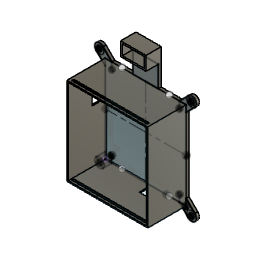
PCBCase (Autodesk Fusion 360 design; units mm, degrees)
Autodesk Fusion 360 part; units mm, degrees
sketch "Sketch1" plane through (0, 0, 0) normal (0, 1, 0) x (1, 0, 0)
  line L0 (0, 0) -> (95, 0)
  line L1 (95, 0) -> (95, -103)
  line L2 (95, -103) -> (7.75, -103)
  line L3 (0, -95.25) -> (0, 0)
  line L4 (0, -103) -> (7.75, -103)
  line L5 (7.75, -103) -> (7.75, -95.25)
  circle A0 centre (7.75, -95.25) radius 2
  line L6 (0, -103) -> (7.75, -103)
  line L7 (0, -103) -> (0, -95.25)
  line L8 (0, -95.25) -> (-10.6066, -105.8566)
  line L9 (7.75, -103) -> (-2.8566, -113.6066)
  line L10 (7.75, -103) -> (19.75, -103) construction
  line L11 (-10.6066, -105.8566) -> (-2.8566, -113.6066)
  circle A1 centre (-6.7316, -109.7316) radius 5.5
  line L12 (95, -51.5) -> (0, -51.5)
  line L13 (47.5, 0) -> (47.5, -103)
  circle A2 centre (-6.7316, -109.7316) radius 2.5
  circle A3 centre (-6.7316, 6.7316) radius 5.5
  circle A4 centre (7.75, -7.75) radius 2
  line L14 (7.75, 0) -> (19.75, 0) construction
  line L15 (0, -7.75) -> (-10.6066, 2.8566)
  line L16 (7.75, 0) -> (-2.8566, 10.6066)
  line L17 (0, 0) -> (0, -7.75)
  line L18 (7.75, 0) -> (7.75, -7.75)
  line L19 (0, 0) -> (7.75, 0)
  circle A5 centre (-6.7316, 6.7316) radius 2.5
  line L20 (0, 0) -> (7.75, 0)
  line L21 (-10.6066, 2.8566) -> (-2.8566, 10.6066)
  line L22 (87.25, -103) -> (75.25, -103) construction
  circle A6 centre (87.25, -95.25) radius 2
  line L23 (87.25, -103) -> (87.25, -95.25)
  line L24 (95, -95.25) -> (105.6066, -105.8566)
  line L25 (105.6066, -105.8566) -> (97.8566, -113.6066)
  circle A7 centre (101.7316, -109.7316) radius 5.5
  line L26 (95, -103) -> (87.25, -103)
  circle A8 centre (101.7316, -109.7316) radius 2.5
  line L27 (95, -103) -> (87.25, -103)
  line L28 (105.6066, 2.8566) -> (97.8566, 10.6066)
  line L29 (87.25, 0) -> (87.25, -7.75)
  line L30 (87.25, 0) -> (75.25, 0) construction
  line L31 (95, 0) -> (87.25, 0)
  line L32 (95, -103) -> (95, -95.25)
  line L33 (95, -7.75) -> (105.6066, 2.8566)
  line L34 (95, 0) -> (95, -7.75)
  line L35 (95, 0) -> (87.25, 0)
  line L36 (87.25, -103) -> (97.8566, -113.6066)
  circle A9 centre (101.7316, 6.7316) radius 2.5
  circle A10 centre (87.25, -7.75) radius 2
  line L37 (87.25, 0) -> (97.8566, 10.6066)
  circle A11 centre (101.7316, 6.7316) radius 5.5
  line L38 (47.5, -103) -> (62.4, -103)
  line L39 (62.4, -103) -> (32.6, -103)
  line L40 (32.6, -103) -> (32.6, -128)
  line L41 (32.6, -128) -> (62.4, -128)
  line L42 (62.4, -128) -> (62.4, -103)
  point P0 (95, 0)
  point P1 (95, -51.5)
  point P2 (95, 0)
  dimension "d1" = 95
  dimension "d2" = 103
  dimension "d3" = 7.75
  dimension "d4" = 7.75
  dimension "d5" = 4
  dimension "d6" = 7.75
  dimension "d7" = 7.75
  dimension "d8" = 15
  dimension "d9" = 135
  dimension "d10" = 135
  dimension "d11" = 15
  dimension "d12" = 11
  dimension "d17" = 5
  dimension "d58" = 14.9
  dimension "d59" = 29.8
  dimension "d60" = 25
  constraint horizontal L0
  constraint vertical L1
  constraint horizontal L2
  constraint vertical L3
  constraint coincident L0.start L3.end
  constraint perpendicular L3 L4
  constraint perpendicular L2 L5
  constraint coincident L5.end A0.centre
  constraint perpendicular L3 L6
  constraint perpendicular L4 L7
  constraint horizontal L10
  constraint midpoint L11 A1.centre
  constraint midpoint L1 P1
  constraint coincident L3 L12.end
  constraint perpendicular L3 L12
  constraint midpoint L0 L13.start
  constraint coincident L2 L13.end
  constraint perpendicular L2 L13
  constraint concentric A1 A2
  constraint symmetric L4.start L12 L0.start
  constraint symmetric L2.end L12 L14.start
  constraint symmetric L5.end L12 A4.centre
  constraint symmetric A0 L12 A4
  constraint symmetric L3.start L12 L15.start
  constraint symmetric L8.end L12 L15.end
  constraint symmetric L9.end L12 L16.end
  constraint symmetric L10.end L12 L14.end
  constraint symmetric A1 L12 A3
  constraint symmetric L12 A2 A5
  constraint symmetric L0.start L13 P2
  constraint symmetric L4.start L13 L1.end
  constraint symmetric L2.end L13 L22.start
  constraint symmetric L5.end L13 A6.centre
  constraint symmetric A0 L13 A6
  constraint symmetric L3.start L13 L24.start
  constraint symmetric L8.end L13 L24.end
  constraint symmetric L9.end L13 L25.end
  constraint symmetric L10.end L13 L22.end
  constraint symmetric A1 L13 A7
  constraint symmetric L12.end L13 P1
  constraint symmetric L13 A2 A8
  constraint symmetric L13 L15.start L33.start
  constraint symmetric L13 L16.end L28.end
  constraint symmetric L13 L15.end L28.start
  constraint symmetric L13 L14.start L29.start
  constraint symmetric L13 A4.centre L29.end
  constraint symmetric L13 L14.end L30.end
  constraint symmetric L13 L0.start P2
  constraint symmetric L13 A3 A11
  constraint symmetric L13 A4 A10
  constraint symmetric L13 A5 A9
  constraint perpendicular L13 L38
  constraint horizontal L39
  constraint vertical L40
  constraint horizontal L41
  constraint vertical L42
  measures "d1" distance of L0.start P0
  measures "d2" distance of L0.start L4.start
  measures "d3" distance of L4.start L2.end
  measures "d4" distance of L2.end L5.end
  measures "d5" diameter of A0
  measures "d6" distance of L4.start L2.end
  measures "d7" distance of L4.start L3.start
  measures "d8" distance of L3.start L8.end
  measures "d9" angle of L3 L8
  measures "d10" angle of L9 L10
  measures "d11" distance of L2.end L9.end
  measures "d12" diameter of A1
  measures "d17" diameter of A2
  measures "d58" distance of L13.end L38.end
  measures "d59" distance of L38.end L39.end
  measures "d60" distance of L38.end L41.end
extrude "Extrude1" add sketch "Sketch1" along normal blind 3.5 contours L0 L3 A3 L15 L16 L17 L19 L20 | L0 L3 L12 L13 L17 L19 L20 | L0 L1 L12 L13 L31 L34 L35 | A3 L15 L16 A5 L21 | A3 L15 L16 A5 L21 | L2 L3 L4 L6 L7 L12 L13 L39 | L0 L1 L31 L33 L34 L35 L37 A11 | L1 L2 L12 L13 L26 L27 L32 L38 L39 | L4 L6 L7 L8 L9 A1 | L28 L33 A9 L37 A11 | L28 L33 A9 L37 A11 | L8 L9 L11 A1 A2 | L8 L9 L11 A1 A2 | L1 L2 L24 A7 L26 L27 L32 L36 | L24 L25 A7 A8 L36 | L24 L25 A7 A8 L36
sketch "Sketch2" plane through (0, 0, 0) normal (0, -1, 0) x (1, 0, 0)
  circle A0 centre (7.75, 7.75) radius 2
  circle A1 centre (87.25, 7.75) radius 2
  circle A2 centre (-6.7316, -6.7316) radius 2.5
  circle A3 centre (101.7316, -6.7316) radius 2.5
  circle A4 centre (87.25, 95.25) radius 2
  circle A5 centre (101.7316, 109.7316) radius 2.5
  circle A6 centre (7.75, 95.25) radius 2
  circle A7 centre (-6.7316, 109.7316) radius 2.5
  line L0 (105.2759, -2.5259) -> (95, 7.75)
  line L1 (95, 7.75) -> (95, 95.25)
  line L2 (95, 95.25) -> (105.2759, 105.5259)
  arc A8 (105.2759, 105.5259) -> (97.5259, 113.2759) centre (101.7316, 109.7316) ccw
  line L3 (97.5259, 113.2759) -> (87.25, 103)
  line L4 (87.25, 103) -> (7.75, 103)
  line L5 (7.75, 103) -> (-2.5259, 113.2759)
  arc A9 (-2.5259, 113.2759) -> (-10.2759, 105.5259) centre (-6.7316, 109.7316) ccw
  line L6 (-10.2759, 105.5259) -> (0, 95.25)
  line L7 (0, 95.25) -> (0, 7.75)
  line L8 (0, 7.75) -> (-10.2759, -2.5259)
  arc A10 (-10.2759, -2.5259) -> (-2.5259, -10.2759) centre (-6.7316, -6.7316) ccw
  line L9 (-2.5259, -10.2759) -> (7.75, 0)
  line L10 (7.75, 0) -> (87.25, 0)
  line L11 (87.25, 0) -> (97.5259, -10.2759)
  arc A11 (97.5259, -10.2759) -> (105.2759, -2.5259) centre (101.7316, -6.7316) ccw
  line L12 (47.5, 103) -> (47.5, 0) construction
  line L13 (0, 51.5) -> (95, 51.5) construction
  line L14 (0, 0) -> (1.5, 0)
  line L15 (1.5, 0) -> (1.5, 103)
  line L16 (1.5, 103) -> (0, 103)
  line L17 (0, 103) -> (0, 0)
  line L18 (95, 103) -> (95, 0)
  line L19 (93.5, 0) -> (93.5, 103)
  line L20 (93.5, 103) -> (95, 103)
  line L21 (95, 0) -> (93.5, 0)
  line L22 (0, 103) -> (95, 103)
  line L23 (95, 103) -> (95, 101.5)
  line L24 (95, 101.5) -> (0, 101.5)
  line L25 (0, 101.5) -> (0, 103)
  line L26 (95, 1.5) -> (0, 1.5)
  line L27 (0, 0) -> (95, 0)
  line L28 (95, 0) -> (95, 1.5)
  line L29 (0, 1.5) -> (0, 0)
  dimension "d22" = 1.5
  dimension "d23" = 103
  dimension "d24" = 95
  dimension "d25" = 1.5
  constraint midpoint L4 L12.start
  constraint midpoint L10 L12.end
  constraint midpoint L7 L13.start
  constraint midpoint L1 L13.end
  constraint horizontal L14
  constraint vertical L15
  constraint horizontal L16
  constraint vertical L17
  constraint coincident L14.start L17.end
  constraint symmetric L12 L14.start L18.end
  constraint symmetric L12 L14.end L19.start
  constraint symmetric L12 L15.end L19.end
  constraint symmetric L12 L16.end L18.start
  constraint horizontal L22
  constraint vertical L23
  constraint horizontal L24
  constraint vertical L25
  constraint symmetric L13 L16.end L14.start
  constraint symmetric L13 L18.start L18.end
  constraint symmetric L13 L23.end L26.start
  constraint symmetric L13 L24.end L26.end
  measures "d22" distance of L14.start L14.end
  measures "d23" distance of L14.start L16.end
  measures "d24" distance of L16.end L18.start
  measures "d25" distance of L16.end L24.end
extrude "Extrude2" add sketch "Sketch2" along normal blind 45 contours L1 L18 L19 L24 L26 | L18 L19 L21 L26 L27 L28 | L10 L15 L19 L26 L27 | L18 L19 L20 L22 L23 L24 | L4 L15 L19 L22 L24 | L7 L15 L17 L24 L26 | L14 L15 L17 L26 L27 L29 | L15 L16 L17 L22 L24 L25
sketch "Sketch3" plane through (0, 0, 0) normal (0, 0, -1) x (1, 0, 0)
  line L0 (7.75, 0) -> (7.75, -3.5)
  line L1 (7.75, -3.5) -> (87.25, -3.5)
  line L2 (87.25, -3.5) -> (87.25, 0)
  line L3 (87.25, 0) -> (95, 0)
  line L4 (95, 0) -> (95, 45)
  line L5 (95, 45) -> (0, 45)
  line L6 (0, 45) -> (0, 0)
  line L7 (0, 0) -> (7.75, 0)
  line L8 (0, 45) -> (0, 42.5)
  line L9 (0, 42.5) -> (3, 42.5)
  line L10 (3, 42.5) -> (92, 42.5)
  line L11 (92, 42.5) -> (92, 40)
  line L12 (92, 40) -> (3, 40)
  line L13 (3, 40) -> (3, 42.5)
  dimension "d28" = 2.5
  dimension "d29" = 3
  dimension "d30" = 89
  dimension "d31" = 2.5
  constraint coincident L5.end L6.start
  constraint perpendicular L5 L8
  constraint perpendicular L8 L9
  constraint horizontal L10
  constraint vertical L11
  constraint horizontal L12
  constraint vertical L13
  measures "d28" distance of L5.end L8.end
  measures "d29" distance of L8.end L9.end
  measures "d30" distance of L9.end L10.end
  measures "d31" distance of L9.end L12.end
extrude "Extrude3" cut sketch "Sketch3" against normal blind 156 contours L10 L11 L12 L13
sketch "Sketch4" plane through (0, 0, 0) normal (0, -1, 0) x (1, 0, 0)
  circle A0 centre (7.75, 95.25) radius 2
  circle A1 centre (87.25, 95.25) radius 2
  circle A2 centre (87.25, 7.75) radius 2
  circle A3 centre (7.75, 7.75) radius 2
  line L0 (93.5, 1.5) -> (93.5, 101.5)
  line L1 (93.5, 101.5) -> (1.5, 101.5)
  line L2 (1.5, 101.5) -> (1.5, 1.5)
  line L3 (1.5, 1.5) -> (93.5, 1.5)
extrude "Extrude5" add sketch "Sketch1" along normal blind 3.5 contours L0 L3 L12 L13 L17 L19 L20
sketch "Sketch5" plane through (0, 3.5, 0) normal (0, 1, 0) x (-1, 0, 0)
  circle A0 centre (-7.75, 95.25) radius 2
  circle A1 centre (6.7316, 109.7316) radius 2.5
  circle A2 centre (-101.7316, -6.7316) radius 2.5
  circle A3 centre (-101.7316, 109.7316) radius 2.5
  circle A4 centre (-87.25, 95.25) radius 2
  circle A5 centre (-7.75, 7.75) radius 2
  circle A6 centre (6.7316, -6.7316) radius 2.5
  circle A7 centre (-87.25, 7.75) radius 2
  line L0 (-95, 7.75) -> (-105.2759, -2.5259)
  arc A8 (-105.2759, -2.5259) -> (-97.5259, -10.2759) centre (-101.7316, -6.7316) ccw
  line L1 (-97.5259, -10.2759) -> (-87.25, 0)
  line L2 (-87.25, 0) -> (-7.75, 0)
  line L3 (-7.75, 0) -> (2.5259, -10.2759)
  arc A9 (2.5259, -10.2759) -> (10.2759, -2.5259) centre (6.7316, -6.7316) ccw
  line L4 (10.2759, -2.5259) -> (0, 7.75)
  line L5 (0, 7.75) -> (0, 95.25)
  line L6 (0, 95.25) -> (10.2759, 105.5259)
  arc A10 (10.2759, 105.5259) -> (2.5259, 113.2759) centre (6.7316, 109.7316) ccw
  line L7 (2.5259, 113.2759) -> (-7.75, 103)
  line L8 (-7.75, 103) -> (-87.25, 103)
  line L9 (-87.25, 103) -> (-97.5259, 113.2759)
  arc A11 (-97.5259, 113.2759) -> (-105.2759, 105.5259) centre (-101.7316, 109.7316) ccw
  line L10 (-105.2759, 105.5259) -> (-95, 95.25)
  line L11 (-95, 95.25) -> (-95, 7.75)
  line L12 (25, 66.4) -> (41.2, 66.4)
  line L13 (41.2, 66.4) -> (41.2, 36.6)
  line L14 (41.2, 36.6) -> (25, 36.6)
  line L15 (25, 36.6) -> (25, 66.4)
  dimension "d48" = 16.2
  dimension "d49" = 29.8
  constraint horizontal L12
  constraint vertical L13
  constraint horizontal L14
  constraint vertical L15
  measures "d48" distance of L12.start L12.end
  measures "d49" distance of L12.start L14.end
extrude "Extrude8" add sketch "Sketch1" along normal blind 3.5 contours L2 L38 L39 L40 L41 L42
sketch "Sketch7" plane through (0, 3.5, 0) normal (0, 1, 0) x (-1, 0, 0)
  line L0 (-62.4, 128) -> (-62.4, 103)
  line L1 (-7.75, 103) -> (-32.6, 103)
  line L2 (-32.6, 103) -> (-32.6, 128)
  line L3 (-32.6, 128) -> (-62.4, 128)
  line L4 (-62.4, 128) -> (-32.6, 128)
  line L5 (-32.6, 128) -> (-32.6, 144.2)
  line L6 (-32.6, 144.2) -> (-62.4, 144.2)
  line L7 (-62.4, 144.2) -> (-62.4, 128)
  circle A0 centre (6.7316, -6.7316) radius 2.5
  circle A1 centre (-7.75, 7.75) radius 2
  line L8 (-87.25, 0) -> (-7.75, 0)
  line L9 (-7.75, 0) -> (2.5259, -10.2759)
  arc A2 (2.5259, -10.2759) -> (10.2759, -2.5259) centre (6.7316, -6.7316) ccw
  line L10 (10.2759, -2.5259) -> (0, 7.75)
  line L11 (0, 7.75) -> (0, 95.25)
  line L12 (0, 95.25) -> (10.2759, 105.5259)
  arc A3 (10.2759, 105.5259) -> (2.5259, 113.2759) centre (6.7316, 109.7316) ccw
  line L13 (2.5259, 113.2759) -> (-7.75, 103)
  line L14 (-62.4, 103) -> (-87.25, 103)
  line L15 (-87.25, 103) -> (-97.5259, 113.2759)
  arc A4 (-97.5259, 113.2759) -> (-105.2759, 105.5259) centre (-101.7316, 109.7316) ccw
  line L16 (-105.2759, 105.5259) -> (-95, 95.25)
  line L17 (-95, 95.25) -> (-95, 7.75)
  line L18 (-95, 7.75) -> (-105.2759, -2.5259)
  arc A5 (-105.2759, -2.5259) -> (-97.5259, -10.2759) centre (-101.7316, -6.7316) ccw
  line L19 (-97.5259, -10.2759) -> (-87.25, 0)
  circle A6 centre (-7.75, 95.25) radius 2
  circle A7 centre (-87.25, 7.75) radius 2
  circle A8 centre (-87.25, 95.25) radius 2
  circle A9 centre (6.7316, 109.7316) radius 2.5
  circle A10 centre (-101.7316, 109.7316) radius 2.5
  circle A11 centre (-101.7316, -6.7316) radius 2.5
  dimension "d63" = 29.8
  dimension "d64" = 16.2
  constraint horizontal L4
  constraint vertical L5
  constraint horizontal L6
  constraint vertical L7
  constraint coincident L0.start L3.end
  measures "d63" distance of L0.start L2.end
  measures "d64" distance of L0.start L6.end
extrude "Extrude9" add sketch "Sketch7" against normal blind 18 contours L3 L4 L5 L6 L7
sketch "Sketch8" plane through (0, -14.5, 0) normal (0, -1, 0) x (1, 0, 0)
  line L0 (62.4, 128) -> (62.4, 144.2)
  line L1 (62.4, 144.2) -> (32.6, 144.2)
  line L2 (32.6, 144.2) -> (32.6, 128)
  line L3 (32.6, 128) -> (62.4, 128)
  line L4 (62.4, 144.2) -> (62.4, 142.2)
  line L5 (62.4, 142.2) -> (60.4, 142.2)
  line L6 (60.4, 142.2) -> (34.6, 142.2)
  line L7 (34.6, 142.2) -> (34.6, 130)
  line L8 (34.6, 130) -> (60.4, 130)
  line L9 (60.4, 130) -> (60.4, 142.2)
  dimension "d67" = 2
  dimension "d68" = 2
  dimension "d69" = 25.8
  dimension "d70" = 12.2
  constraint coincident L0.end L1.start
  constraint perpendicular L1 L4
  constraint perpendicular L4 L5
  constraint horizontal L6
  constraint vertical L7
  constraint horizontal L8
  constraint vertical L9
  measures "d67" distance of L0.end L4.end
  measures "d68" distance of L4.end L5.end
  measures "d69" distance of L5.end L6.end
  measures "d70" distance of L5.end L8.end
extrude "Extrude10" cut sketch "Sketch8" against normal blind 15 contours L6 L7 L8 L9
sketch "Sketch9" plane through (0, 0, 0) normal (-1, 0, 0) x (0, -1, 0)
  line L0 (-3.5, 95.25) -> (-3.5, 7.75)
  line L1 (-3.5, 7.75) -> (0, 7.75)
  line L2 (0, 7.75) -> (0, 0)
  line L3 (0, 0) -> (45, 0)
  line L4 (45, 0) -> (45, 103)
  line L5 (45, 103) -> (0, 103)
  line L6 (0, 103) -> (0, 95.25)
  line L7 (0, 95.25) -> (-3.5, 95.25)
  line L8 (0, 103) -> (0, 90.5)
  line L9 (0, 90.5) -> (8.6, 90.5)
  line L10 (8.6, 90.5) -> (17, 90.5)
  line L11 (17, 90.5) -> (17, 63.5)
  line L12 (17, 63.5) -> (8.6, 63.5)
  line L13 (8.6, 63.5) -> (8.6, 90.5)
  dimension "d73" = 12.5
  dimension "d74" = 8.6
  dimension "d75" = 8.4
  dimension "d76" = 27
  constraint coincident L5.end L6.start
  constraint perpendicular L7 L8
  constraint perpendicular L8 L9
  constraint horizontal L10
  constraint vertical L11
  constraint horizontal L12
  constraint vertical L13
  measures "d73" distance of L5.end L8.end
  measures "d74" distance of L8.end L9.end
  measures "d75" distance of L9.end L10.end
  measures "d76" distance of L9.end L12.end
extrude "Extrude11" cut sketch "Sketch9" against normal blind 6 contours L10 L11 L12 L13
sketch "Sketch10" plane through (0, 0, 0) normal (0, 0, -1) x (1, 0, 0)
  line L0 (7.75, -3.5) -> (87.25, -3.5)
  line L1 (87.25, -3.5) -> (87.25, 0)
  line L2 (87.25, 0) -> (95, 0)
  line L3 (95, 0) -> (95, 45)
  line L4 (95, 45) -> (0, 45)
  line L5 (0, 45) -> (0, 0)
  line L6 (0, 0) -> (7.75, 0)
  line L7 (7.75, 0) -> (7.75, -3.5)
  line L8 (92, 42.5) -> (92, 40)
  line L9 (92, 40) -> (3, 40)
  line L10 (3, 40) -> (3, 42.5)
  line L11 (3, 42.5) -> (92, 42.5)
  line L12 (95, 0) -> (84, 0)
  line L13 (84, 0) -> (84, 1.4)
  line L14 (84, 1.4) -> (55, 1.4)
  line L15 (55, 1.4) -> (55, 15)
  line L16 (55, 15) -> (84, 15)
  line L17 (84, 15) -> (84, 1.4)
  dimension "d79" = 11
  dimension "d80" = 1.4
  dimension "d81" = 29
  dimension "d82" = 13.6
  constraint coincident L2.end L3.start
  constraint perpendicular L1 L12
  constraint vertical L13
  constraint horizontal L14
  constraint vertical L15
  constraint horizontal L16
  constraint vertical L17
  measures "d79" distance of L2.end L12.end
  measures "d80" distance of L12.end L13.end
  measures "d81" distance of L13.end L14.end
  measures "d82" distance of L13.end L16.end
extrude "Extrude12" cut sketch "Sketch10" against normal blind 10 contours L14 L15 L16 L17
sketch "Sketch11" plane through (0, 0, 0) normal (0, 0, -1) x (1, 0, 0)
  line L0 (55, 1.4) -> (55, 15)
  line L1 (55, 15) -> (84, 15)
  line L2 (84, 15) -> (84, 1.4)
  line L3 (84, 1.4) -> (55, 1.4)
  line L4 (7.75, -3.5) -> (87.25, -3.5)
  line L5 (87.25, -3.5) -> (87.25, 0)
  line L6 (87.25, 0) -> (95, 0)
  line L7 (95, 0) -> (95, 45)
  line L8 (95, 45) -> (0, 45)
  line L9 (0, 45) -> (0, 0)
  line L10 (0, 0) -> (7.75, 0)
  line L11 (7.75, 0) -> (7.75, -3.5)
  line L12 (92, 42.5) -> (92, 40)
  line L13 (92, 40) -> (3, 40)
  line L14 (3, 40) -> (3, 42.5)
  line L15 (3, 42.5) -> (92, 42.5)
  line L16 (95, 0) -> (72, 0)
  dimension "d85" = 23
  constraint coincident L6.end L7.start
  constraint perpendicular L0 L16
  measures "d85" distance of L6.end L16.end
equation "d3 = screwHolePlacement"
equation "d5 = screwHoleDiameter"
equation "d6 = screwHolePlacement"
equation "d7 = screwHolePlacement"
equation "d8 = cornerRectangleLength"
equation "d11 = cornerRectangleLength"
equation "d12 = cornerCircleDiameter"
equation "screwHolePlacement = 7.75 mm"
equation "cornerCircleDiameter = 11 mm"
equation "cornerRectangleLength = 15 mm"
equation "screwHoleDiameter = 4 mm"
equation "d17 = cornerHoleDiameter"
equation "cornerHoleDiameter = 5 mm"
equation "d19 = boardThickness"
equation "boardThickness = 3.5 mm"
